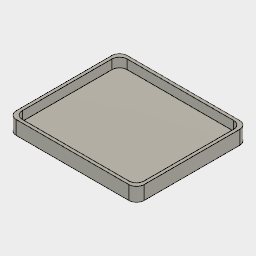
CaseV2 Top v4 (Autodesk Fusion 360 design; units mm, degrees)
Autodesk Fusion 360 part; units mm, degrees
note: some values were not read from the file. Set by a fixed rule: which face or edge a step refers to.
sketch "Sketch1" plane through (0, 0, 0) normal (0, 1, 0) x (1, 0, 0)
  line L0 (41.5, -36) -> (-41.5, -36)
  line L1 (-41.5, -36) -> (-41.5, 36)
  line L2 (-41.5, 36) -> (41.5, 36)
  line L3 (41.5, 36) -> (41.5, -36)
  line L4 (41.5, -36) -> (-41.5, 36) construction
  line L5 (-41.5, -36) -> (41.5, 36) construction
  dimension "d1" = 83
  dimension "d2" = 72
  measures "d1" distance of L1.end L2.end
  measures "d2" distance of L0.end L1.end
extrude "Extrude1" add sketch "Sketch1" along normal blind 9
shell "Shell1" thickness 2 removed faces 1 at (-13.8333, 9, 12)
extrude "Extrude2" add 1 faces at (13.1667, 2, 11.3333) along direction (0, 1, 0) blind 1
fillet "Fillet1" chord length 7 8 edges at (-41.5, 4.5, 36) (41.5, 4.5, 36) (39.5, 6, -34) (39.5, 6, 34) (-41.5, 4.5, -36) (-39.5, 6, -34) (41.5, 4.5, -36) (-39.5, 6, 34)
sketch "Sketch2" plane through (0, 0, 0) normal (0, -1, 0) x (1, 0, 0)
  spline S0 degree 3 poles (41.5, -31.0503) (41.5, -31.7038) (41.3706, -32.351) (40.8647, -33.5648) (40.4904, -34.1183) (39.5647, -35.0274) (39.0293, -35.3814) (37.8418, -35.8724) (37.1992, -36) (36.5503, -36) knots 0 0 0 0 0.196069 0.196069 0.394523 0.394523 0.585313 0.585313 0.779995 0.779995 0.779995 0.779995
  line L0 (41.5, -31.0503) -> (41.5, 31.0503)
  spline S1 degree 3 poles (36.5503, 36) (37.2038, 36) (37.851, 35.8706) (39.0648, 35.3647) (39.6183, 34.9904) (40.5274, 34.0647) (40.8814, 33.5293) (41.3724, 32.3418) (41.5, 31.6992) (41.5, 31.0503) knots 0 0 0 0 0.196069 0.196069 0.394523 0.394523 0.585313 0.585313 0.779995 0.779995 0.779995 0.779995
  line L1 (36.5503, 36) -> (-36.5503, 36)
  spline S2 degree 3 poles (-41.5, 31.0503) (-41.5, 31.7038) (-41.3706, 32.351) (-40.8647, 33.5648) (-40.4904, 34.1183) (-39.5647, 35.0274) (-39.0293, 35.3814) (-37.8418, 35.8724) (-37.1992, 36) (-36.5503, 36) knots 0 0 0 0 0.196069 0.196069 0.394523 0.394523 0.585313 0.585313 0.779995 0.779995 0.779995 0.779995
  line L2 (-41.5, 31.0503) -> (-41.5, -31.0503)
  spline S3 degree 3 poles (-36.5503, -36) (-37.2038, -36) (-37.851, -35.8706) (-39.0648, -35.3647) (-39.6183, -34.9904) (-40.5274, -34.0647) (-40.8814, -33.5293) (-41.3724, -32.3418) (-41.5, -31.6992) (-41.5, -31.0503) knots 0 0 0 0 0.196069 0.196069 0.394523 0.394523 0.585313 0.585313 0.779995 0.779995 0.779995 0.779995
  line L3 (-36.5503, -36) -> (36.5503, -36)
  spline S4 degree 3 poles (-28.6503, 0.3923) (-28.6503, -0.6616) (-29.3704, -1.6133) (-30.5147, -1.6133) knots 0 0 0 0 1 1 1 1
  spline S5 degree 3 poles (-30.5147, -1.6133) (-31.6716, -1.6133) (-32.4044, -0.6489) (-32.4044, 0.4179) knots 0 0 0 0 1 1 1 1
  line L4 (-32.4044, 0.4179) -> (-32.4044, 0.4438)
  spline S6 degree 3 poles (-32.4044, 0.4438) (-32.4044, 1.4981) (-31.6845, 2.4493) (-30.5403, 2.4493) knots 0 0 0 0 1 1 1 1
  spline S7 degree 3 poles (-30.5403, 2.4493) (-29.3831, 2.4493) (-28.6503, 1.485) (-28.6503, 0.4179) knots 0 0 0 0 1 1 1 1
  line L5 (-28.6503, 0.4179) -> (-28.6503, 0.3923)
  spline S8 degree 3 poles (-30.5147, 5.1107) (-33.2914, 5.1107) (-35.4386, 3.0278) (-35.4386, 0.4179) knots 0 0 0 0 1 1 1 1
  line L6 (-35.4386, 0.4179) -> (-35.4386, 0.3923)
  spline S9 degree 3 poles (-35.4386, 0.3923) (-35.4386, -2.2172) (-33.3171, -4.2745) (-30.5403, -4.2745) knots 0 0 0 0 1 1 1 1
  spline S10 degree 3 poles (-30.5403, -4.2745) (-27.7633, -4.2745) (-25.6164, -2.1918) (-25.6164, 0.4179) knots 0 0 0 0 1 1 1 1
  line L7 (-25.6164, 0.4179) -> (-25.6164, 0.4438)
  spline S11 degree 3 poles (-25.6164, 0.4438) (-25.6164, 3.0537) (-27.7377, 5.1107) (-30.5147, 5.1107) knots 0 0 0 0 1 1 1 1
  spline S12 degree 3 poles (-20.255, -1.5744) (-21.2449, -1.5744) (-21.9391, -0.7517) (-21.9391, 0.418) knots 0 0 0 0 1 1 1 1
  line L8 (-21.9391, 0.418) -> (-21.9391, 0.4437)
  spline S13 degree 3 poles (-21.9391, 0.4437) (-21.9391, 1.5238) (-21.2707, 2.4108) (-20.255, 2.4108) knots 0 0 0 0 1 1 1 1
  spline S14 degree 3 poles (-20.255, 2.4108) (-19.4321, 2.4108) (-18.9565, 1.9609) (-18.6224, 1.3182) knots 0 0 0 0 1 1 1 1
  line L9 (-18.6224, 1.3182) -> (-16.1409, 2.7708)
  spline S15 degree 3 poles (-16.1409, 2.7708) (-16.8995, 4.1464) (-18.2364, 5.1107) (-20.2165, 5.1107) knots 0 0 0 0 1 1 1 1
  spline S16 degree 3 poles (-20.2165, 5.1107) (-22.9033, 5.1107) (-24.9988, 3.1052) (-24.9988, 0.418) knots 0 0 0 0 1 1 1 1
  line L10 (-24.9988, 0.418) -> (-24.9988, 0.3923)
  spline S17 degree 3 poles (-24.9988, 0.3923) (-24.9988, -2.3972) (-22.8263, -4.2745) (-20.3322, -4.2745) knots 0 0 0 0 1 1 1 1
  spline S18 degree 3 poles (-20.3322, -4.2745) (-18.0952, -4.2745) (-16.8353, -3.1816) (-16.0768, -1.8445) knots 0 0 0 0 1 1 1 1
  line L11 (-16.0768, -1.8445) -> (-18.5579, -0.4432)
  spline S19 degree 3 poles (-18.5579, -0.4432) (-18.9307, -1.1117) (-19.4064, -1.5744) (-20.255, -1.5744) knots 0 0 0 0 1 1 1 1
  spline S20 degree 3 poles (-11.2165, -1.5744) (-12.2065, -1.5744) (-12.9007, -0.7517) (-12.9007, 0.418) knots 0 0 0 0 1 1 1 1
  line L12 (-12.9007, 0.418) -> (-12.9007, 0.4437)
  spline S21 degree 3 poles (-12.9007, 0.4437) (-12.9007, 1.5238) (-12.2322, 2.4108) (-11.2165, 2.4108) knots 0 0 0 0 1 1 1 1
  spline S22 degree 3 poles (-11.2165, 2.4108) (-10.3937, 2.4108) (-9.9181, 1.9609) (-9.5836, 1.3182) knots 0 0 0 0 1 1 1 1
  line L13 (-9.5836, 1.3182) -> (-7.1025, 2.7708)
  spline S23 degree 3 poles (-7.1025, 2.7708) (-7.861, 4.1464) (-9.198, 5.1107) (-11.178, 5.1107) knots 0 0 0 0 1 1 1 1
  spline S24 degree 3 poles (-11.178, 5.1107) (-13.8649, 5.1107) (-15.9605, 3.1052) (-15.9605, 0.418) knots 0 0 0 0 1 1 1 1
  line L14 (-15.9605, 0.418) -> (-15.9605, 0.3923)
  spline S25 degree 3 poles (-15.9605, 0.3923) (-15.9605, -2.3972) (-13.7879, -4.2745) (-11.2938, -4.2745) knots 0 0 0 0 1 1 1 1
  spline S26 degree 3 poles (-11.2938, -4.2745) (-9.0567, -4.2745) (-7.7969, -3.1816) (-7.0384, -1.8445) knots 0 0 0 0 1 1 1 1
  line L15 (-7.0384, -1.8445) -> (-9.5195, -0.4432)
  spline S27 degree 3 poles (-9.5195, -0.4432) (-9.8923, -1.1117) (-10.368, -1.5744) (-11.2165, -1.5744) knots 0 0 0 0 1 1 1 1
  spline S28 degree 3 poles (-0.6999, -0.0703) (-0.6999, -1.163) (-1.2784, -1.6005) (-2.0885, -1.6005) knots 0 0 0 0 1 1 1 1
  spline S29 degree 3 poles (-2.0885, -1.6005) (-2.8983, -1.6005) (-3.4769, -1.1246) (-3.4769, -0.0062) knots 0 0 0 0 1 1 1 1
  line L16 (-3.4769, -0.0062) -> (-3.4769, 4.9177)
  line L17 (-3.4769, 4.9177) -> (-6.5367, 4.9177)
  line L18 (-6.5367, 4.9177) -> (-6.5367, -0.0449)
  spline S30 degree 3 poles (-6.5367, -0.0449) (-6.5367, -3.0273) (-4.8011, -4.2615) (-2.1142, -4.2615) knots 0 0 0 0 1 1 1 1
  spline S31 degree 3 poles (-2.1142, -4.2615) (0.5728, -4.2615) (2.3598, -3.0531) (2.3598, 0.0196) knots 0 0 0 0 1 1 1 1
  line L19 (2.3598, 0.0196) -> (2.3598, 4.9177)
  line L20 (2.3598, 4.9177) -> (-0.6999, 4.9177)
  line L21 (-0.6999, 4.9177) -> (-0.6999, -0.0703)
  line L22 (6.3199, 4.9177) -> (3.3114, 4.9177)
  line L23 (3.3114, 4.9177) -> (3.3114, -4.0816)
  line L24 (3.3114, -4.0816) -> (10.5496, -4.0816)
  line L25 (10.5496, -4.0816) -> (10.5496, -1.5104)
  line L26 (10.5496, -1.5104) -> (6.3199, -1.5104)
  line L27 (6.3199, -1.5104) -> (6.3199, 4.9177)
  line L28 (32.4458, 4.9177) -> (31.173, 0.598)
  line L29 (31.173, 0.598) -> (29.7201, 4.9435)
  line L30 (29.7201, 4.9435) -> (27.1234, 4.9435)
  line L31 (27.1234, 4.9435) -> (25.6706, 0.598)
  line L32 (25.6706, 0.598) -> (24.3976, 4.9177)
  line L33 (24.3976, 4.9177) -> (21.2478, 4.9177)
  line L34 (21.2478, 4.9177) -> (24.1919, -4.1459)
  line L35 (24.1919, -4.1459) -> (26.8146, -4.1459)
  line L36 (26.8146, -4.1459) -> (28.3959, 0.3281)
  line L37 (28.3959, 0.3281) -> (29.9772, -4.1459)
  line L38 (29.9772, -4.1459) -> (32.5999, -4.1459)
  line L39 (32.5999, -4.1459) -> (35.5441, 4.9177)
  line L40 (35.5441, 4.9177) -> (32.4458, 4.9177)
  spline S32 degree 3 poles (11.6084, 6.4606) (12.7221, 7.7211) (15.5471, 8.6939) (17.4146, 8.2202) knots 0 0 0 0 1 1 1 1
  spline S33 degree 3 poles (17.4146, 8.2202) (17.8157, 8.1185) (18.1065, 8.137) (18.2489, 8.5258) knots 0 0 0 0 1 1 1 1
  spline S34 degree 3 poles (18.2489, 8.5258) (18.3911, 8.9148) (18.1915, 9.3456) (17.8028, 9.488) knots 0 0 0 0 1 1 1 1
  spline S35 degree 3 poles (17.8028, 9.488) (15.3372, 10.3906) (11.7721, 9.0227) (10.4633, 7.2884) knots 0 0 0 0 1 1 1 1
  spline S36 degree 3 poles (10.4633, 7.2884) (10.2139, 6.9575) (10.2801, 6.4876) (10.6103, 6.2381) knots 0 0 0 0 1 1 1 1
  spline S37 degree 3 poles (10.6103, 6.2381) (10.7456, 6.1356) (10.9046, 6.0867) (11.0622, 6.0869) knots 0 0 0 0 1 1 1 1
  spline S38 degree 3 poles (11.0622, 6.0869) (11.2894, 6.0871) (11.4464, 6.2773) (11.6084, 6.4606) knots 0 0 0 0 1 1 1 1
  spline S39 degree 3 poles (12.0493, 3.5375) (12.7446, 4.7071) (13.8526, 5.5352) (15.1692, 5.8696) knots 0 0 0 0 1 1 1 1
  spline S40 degree 3 poles (15.1692, 5.8696) (16.4863, 6.2046) (17.8554, 6.0058) (19.0249, 5.3103) knots 0 0 0 0 1 1 1 1
  spline S41 degree 3 poles (19.0249, 5.3103) (19.3802, 5.0986) (19.8405, 5.2158) (20.0525, 5.5717) knots 0 0 0 0 1 1 1 1
  spline S42 degree 3 poles (20.0525, 5.5717) (20.2643, 5.9276) (20.1473, 6.3879) (19.7913, 6.5995) knots 0 0 0 0 1 1 1 1
  spline S43 degree 3 poles (19.7913, 6.5995) (18.2773, 7.4999) (16.5052, 7.7567) (14.7999, 7.3236) knots 0 0 0 0 1 1 1 1
  spline S44 degree 3 poles (14.7999, 7.3236) (13.0949, 6.8904) (11.6601, 5.8181) (10.76, 4.3042) knots 0 0 0 0 1 1 1 1
  spline S45 degree 3 poles (10.76, 4.3042) (10.5486, 3.9481) (10.6654, 3.4879) (11.0212, 3.2761) knots 0 0 0 0 1 1 1 1
  spline S46 degree 3 poles (11.0212, 3.2761) (11.1362, 3.2078) (11.2615, 3.1736) (11.3862, 3.1707) knots 0 0 0 0 1 1 1 1
  spline S47 degree 3 poles (11.3862, 3.1707) (11.6483, 3.1644) (11.9059, 3.2962) (12.0493, 3.5375) knots 0 0 0 0 1 1 1 1
  spline S48 degree 3 poles (16.1992, 1.5989) (15.4612, 1.4951) (14.7786, 2.0092) (14.6747, 2.7472) knots 0 0 0 0 1 1 1 1
  spline S49 degree 3 poles (14.6747, 2.7472) (14.571, 3.4856) (15.0853, 4.1681) (15.8234, 4.2718) knots 0 0 0 0 1 1 1 1
  spline S50 degree 3 poles (15.8234, 4.2718) (16.5612, 4.3756) (17.2436, 3.8614) (17.3475, 3.1232) knots 0 0 0 0 1 1 1 1
  spline S51 degree 3 poles (17.3475, 3.1232) (17.4512, 2.385) (16.9372, 1.7026) (16.1992, 1.5989) knots 0 0 0 0 1 1 1 1
  spline S52 degree 3 poles (16.6793, -0.2959) (16.3351, -0.2959) (16.0552, -0.016) (16.0552, 0.3281) knots 0 0 0 0 1 1 1 1
  spline S53 degree 3 poles (16.0552, 0.3281) (16.0552, 0.672) (16.3351, 0.9521) (16.6793, 0.9521) knots 0 0 0 0 1 1 1 1
  spline S54 degree 3 poles (16.6793, 0.9521) (17.0233, 0.9521) (17.303, 0.672) (17.303, 0.3281) knots 0 0 0 0 1 1 1 1
  spline S55 degree 3 poles (17.303, 0.3281) (17.303, -0.016) (17.0233, -0.2959) (16.6793, -0.2959) knots 0 0 0 0 1 1 1 1
  spline S56 degree 3 poles (16.6918, 5.0206) (13.9152, 5.0206) (11.768, 2.9377) (11.768, 0.3278) knots 0 0 0 0 1 1 1 1
  line L41 (11.768, 0.3278) -> (11.768, 0.3024)
  spline S57 degree 3 poles (11.768, 0.3024) (11.768, -2.3074) (13.8893, -4.3646) (16.6662, -4.3646) knots 0 0 0 0 1 1 1 1
  spline S58 degree 3 poles (16.6662, -4.3646) (19.4431, -4.3646) (21.5901, -2.282) (21.5901, 0.3278) knots 0 0 0 0 1 1 1 1
  line L42 (21.5901, 0.3278) -> (21.5901, 0.3538)
  spline S59 degree 3 poles (21.5901, 0.3538) (21.5901, 2.9637) (19.4687, 5.0206) (16.6918, 5.0206) knots 0 0 0 0 1 1 1 1
extrude "Extrude3" cut sketch "Sketch2" against normal blind 1 contours S8 L6 S9 S10 L7 S11 | S12 L8 S13 S14 L9 S15 S16 L10 S17 S18 L11 S19 | S20 L12 S21 S22 L13 S23 S24 L14 S25 S26 L15 S27 | S28 S29 L16 L17 L18 S30 S31 L19 L20 L21 | L22 L23 L24 L25 L26 L27 | L28 L29 L30 L31 L32 L33 L34 L35 L36 L37 L38 L39 L40 | S32 S33 S34 S35 S36 S37 S38 | S39 S40 S41 S42 S43 S44 S45 S46 S47 | S56 L41 S57 S58 L42 S59
